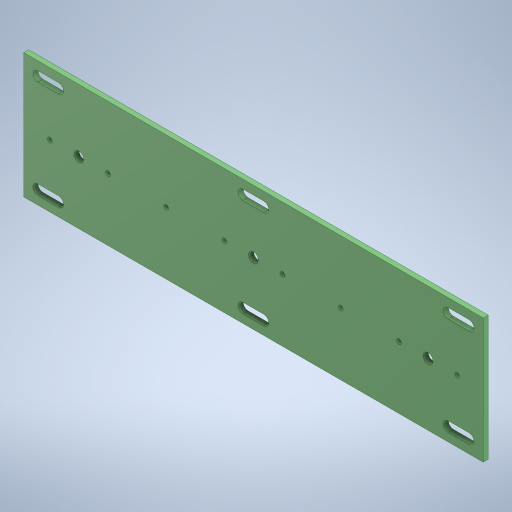
# Autodesk Inventor part: PCB SiPM 8CH larga
Saved by Autodesk Inventor 2024.2 (Build 282272000, 272)
## iProperties
Created: 2024-08-30
Part Number: PCB SiPM 8CH larga
Material: Phenolic Resin
Document SubType Name: Modeling
Designer: ja.restrepo1
Density: 1.38 g/cm^3
Appearance: Smooth - Dark Forest Green
Author: ja.restrepo1
Autodesk Inventor part; units mm, degrees
ref_plane "YZ Plane" through (0, 0, 0) normal (1, 0, 0) x (0, 1, 0)
ref_plane "XZ Plane" through (0, 0, 0) normal (0, 1, 0) x (-1, 0, 0)
ref_plane "XY Plane" through (0, 0, 0) normal (0, 0, 1) x (1, 0, 0)
sketch "Sketch1" plane through (0, 0, 0) normal (0, 0, 1) x (1, 0, 0)
  line L0 (-75, 20.4) -> (75, 20.4)
  line L1 (75, 20.4) -> (75, -20.4)
  line L2 (75, -20.4) -> (-75, -20.4)
  line L3 (-75, -20.4) -> (-75, 20.4)
  circle A0 centre (-57, 0) radius 1.6
  circle A1 centre (0, 0) radius 1.6
  circle A2 centre (57, 0) radius 1.6
  line L4 (-70.4, 16) -> (-63.6, 16) construction
  line L5 (-70.4, 14.4) -> (-63.6, 14.4)
  line L6 (-63.6, 17.6) -> (-70.4, 17.6)
  arc A3 (-70.4, 17.6) -> (-70.4, 14.4) centre (-70.4, 16) ccw
  arc A4 (-63.6, 14.4) -> (-63.6, 17.6) centre (-63.6, 16) ccw
  line L7 (-3.4, 16) -> (3.4, 16) construction
  line L8 (-3.4, 14.4) -> (3.4, 14.4)
  line L9 (3.4, 17.6) -> (-3.4, 17.6)
  arc A5 (-3.4, 17.6) -> (-3.4, 14.4) centre (-3.4, 16) ccw
  arc A6 (3.4, 14.4) -> (3.4, 17.6) centre (3.4, 16) ccw
  line L10 (-70.4, -16) -> (-63.6, -16) construction
  line L11 (-70.4, -17.6) -> (-63.6, -17.6)
  line L12 (-63.6, -14.4) -> (-70.4, -14.4)
  arc A7 (-70.4, -14.4) -> (-70.4, -17.6) centre (-70.4, -16) ccw
  arc A8 (-63.6, -17.6) -> (-63.6, -14.4) centre (-63.6, -16) ccw
  line L13 (-3.4, -16) -> (3.4, -16) construction
  line L14 (-3.4, -17.6) -> (3.4, -17.6)
  line L15 (3.4, -14.4) -> (-3.4, -14.4)
  arc A9 (-3.4, -14.4) -> (-3.4, -17.6) centre (-3.4, -16) ccw
  arc A10 (3.4, -17.6) -> (3.4, -14.4) centre (3.4, -16) ccw
  line L16 (63.6, 16) -> (70.4, 16) construction
  line L17 (63.6, 14.4) -> (70.4, 14.4)
  line L18 (70.4, 17.6) -> (63.6, 17.6)
  arc A11 (63.6, 17.6) -> (63.6, 14.4) centre (63.6, 16) ccw
  arc A12 (70.4, 14.4) -> (70.4, 17.6) centre (70.4, 16) ccw
  line L19 (63.6, -16) -> (70.4, -16) construction
  line L20 (63.6, -17.6) -> (70.4, -17.6)
  line L21 (70.4, -14.4) -> (63.6, -14.4)
  arc A13 (63.6, -14.4) -> (63.6, -17.6) centre (63.6, -16) ccw
  arc A14 (70.4, -17.6) -> (70.4, -14.4) centre (70.4, -16) ccw
  line L22 (67, 16) -> (67, -16) construction
  circle A15 centre (-66.5, 0) radius 0.75
  circle A16 centre (-47.5, 0) radius 0.75
  circle A17 centre (-28.5, 0) radius 0.75
  circle A18 centre (-9.5, 0) radius 0.75
  circle A19 centre (9.5, 0) radius 0.75
  circle A20 centre (28.5, 0) radius 0.75
  circle A21 centre (47.5, 0) radius 0.75
  circle A22 centre (66.5, 0) radius 0.75
  line L23 (-9.5, 0) -> (9.5, 0) construction
  point P0 (-75, 0)
  point P1 (0, 20.4)
  point P2 (-67, 16)
  point P3 (0, 16)
  point P4 (-67, -16)
  point P5 (0, -16)
  point P6 (67, 0)
  dimension "d0" = 150
  dimension "d1" = 40.8
  dimension "d2" = 3.2
  dimension "d3" = 57
  dimension "d4" = 57
  dimension "d5" = 6.8
  dimension "d6" = 3.2
  dimension "d7" = 6.8
  dimension "d8" = 3.2
  dimension "d9" = 6.8
  dimension "d10" = 3.2
  dimension "d11" = 6.8
  dimension "d12" = 3.2
  dimension "d13" = 6.8
  dimension "d14" = 3.2
  dimension "d15" = 6.8
  dimension "d16" = 3.2
  dimension "d17" = 4.6
  dimension "d18" = 32
  dimension "d19" = 67
  dimension "d20" = 1.5
  dimension "d21" = 1.5
  dimension "d22" = 1.5
  dimension "d23" = 1.5
  dimension "d24" = 1.5
  dimension "d25" = 1.5
  dimension "d26" = 1.5
  dimension "d27" = 1.5
  dimension "d28" = 19
  dimension "d29" = 19
  dimension "d30" = 19
  dimension "d31" = 19
  dimension "d32" = 19
  dimension "d33" = 19
  dimension "d34" = 19
  constraints: 60 end point, 24 point on circle, 24 tangent, 23 centre point, 16 horizontal alignment, 10 midpoint, 8 horizontal, 8 parallel, 5 vertical alignment, 3 coincident, 2 equal radius, 2 perpendicular
  measures "d0" distance of L0.start L0.end
  measures "d1" distance of L2.end L0.start
  measures "d2" diameter of A0
  measures "d3" distance of point (0, 0) A0.centre
  measures "d4" distance of A2.centre A1.centre
  measures "d5" distance of L4.start L4.end
  measures "d6" diameter of A4
  measures "d7" distance of L7.start L7.end
  measures "d8" diameter of A6
  measures "d9" distance of L10.start L10.end
  measures "d10" diameter of A8
  measures "d11" distance of L13.start L13.end
  measures "d12" diameter of A10
  measures "d13" distance of L16.start L16.end
  measures "d14" diameter of A12
  measures "d15" distance of L19.start L19.end
  measures "d16" diameter of A14
  measures "d17" distance from line of L16.end L1
  measures "d18" distance of L22.end L22.start
  measures "d19" distance of point (-67, 16) point (0, 16)
  measures "d20" diameter of A15
  measures "d21" diameter of A16
  measures "d22" diameter of A17
  measures "d23" diameter of A18
  measures "d24" diameter of A19
  measures "d25" diameter of A20
  measures "d26" diameter of A21
  measures "d27" diameter of A22
  measures "d28" distance of L23.end L23.start
  measures "d29" distance of A20.centre L23.end
  measures "d30" distance of A21.centre A20.centre
  measures "d31" distance of A22.centre A21.centre
  measures "d32" distance of L23.start A17.centre
  measures "d33" distance of A17.centre A16.centre
  measures "d34" distance of A16.centre A15.centre
extrude "Cuerpo IC SiPM" add sketch "Sketch1" along normal mid plane 1.6
equation "\"d4\" = d3"
equation "\"d29\" = d28"
equation "\"d30\" = d28"
equation "\"d31\" = d28"
equation "\"d32\" = d28"
equation "\"d33\" = d28"
equation "\"d34\" = d28"
body "Solid1"
